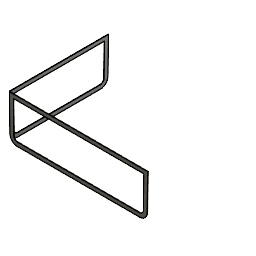
Hardcase_Gridfinity_Perimeter_Template (Autodesk Fusion 360 design; units mm, degrees)
part number: 2026-06-07-12-46-21-203
part number: 2026-06-07-12-46-21-213
Autodesk Fusion 360 part; units mm, degrees
sketch "FRONT" plane through (0, 0, 0) normal (0, 0, 1) x (1, 0, 0)
  line L0 (0, 0) -> (0, 110) construction
  line L1 (0, 110) -> (1.5933, 18.7175)
  line L2 (0, 110) -> (103.8151, 110) construction
  line L3 (20.6404, 0) -> (329.3596, 0)
  line L4 (350, 0) -> (350, 110) construction
  line L5 (350, 110) -> (348.4067, 18.7175)
  line L6 (350, 110) -> (486.4264, 110) construction
  line L7 (350, 110) -> (375.4, 110)
  line L8 (375.4, 110) -> (375.4, -25.4)
  line L9 (375.4, -25.4) -> (-25.4, -25.4)
  line L10 (-25.4, -25.4) -> (-25.4, 110)
  line L11 (-25.4, 110) -> (0, 110)
  arc A0 (1.5933, 18.7175) -> (20.6404, 0) centre (20.6404, 19.05) ccw
  arc A1 (329.3596, 0) -> (348.4067, 18.7175) centre (329.3596, 19.05) ccw
  line L12 (350, 110) -> (0, 110)
  line L13 (339.8239, 100) -> (10.1761, 100)
  line L14 (10.1761, 100) -> (11.5918, 18.8921)
  arc A2 (11.5918, 18.8921) -> (20.6404, 10) centre (20.6404, 19.05) ccw
  line L15 (20.6404, 10) -> (329.3596, 10)
  arc A3 (329.3596, 10) -> (338.4082, 18.8921) centre (329.3596, 19.05) ccw
  line L16 (339.8239, 100) -> (338.4082, 18.8921)
  dimension "d15" = 110
  dimension "d16" = 89
  dimension "d17" = 350
  dimension "d18" = 110
  dimension "d19" = 91
  dimension "d20" = 25.4
  dimension "d21" = 135.4
  dimension "d22" = 400.8
  dimension "d23" = 135.4
  dimension "d24" = 19.05
  constraint coincident L0.start origin
  constraint vertical L0
  constraint horizontal L2
  constraint perpendicular L0 L3
  constraint perpendicular L3 L4
  constraint horizontal L6
  constraint perpendicular L4 L7
  constraint perpendicular L6 L8
  constraint perpendicular L8 L9
  constraint perpendicular L9 L10
  constraint coincident L0.start L3
  constraint tangent L1 A0
  constraint tangent L3 A0
  constraint coincident L4.start L3
  constraint tangent L3 A1
  constraint tangent L5 A1
  constraint equal A0 A1
  measures "d15" distance of L0.start L0.end
  measures "d16" angle of L1 L2
  measures "d17" distance of L0.start L4.start
  measures "d18" distance of L4.start L4.end
  measures "d19" angle of L5 L6
  measures "d20" distance of L4.end L7.end
  measures "d21" distance of L7.end L8.end
  measures "d22" distance of L8.end L9.end
  measures "d23" distance of L9.end L10.end
  measures "d24" radius of A0
sketch "SIDE" plane through (0, 0, 0) normal (1, 0, 0) x (0, 0, -1)
  line L0 (0, 0) -> (0, 110) construction
  line L1 (20.6404, 0) -> (229.3596, 0)
  line L2 (250, 0) -> (250, 110) construction
  line L3 (250, 110) -> (248.4067, 18.7175)
  line L4 (250, 110) -> (374.6664, 110) construction
  line L5 (0, 110) -> (1.5933, 18.7175)
  line L6 (0, 110) -> (107.9664, 110) construction
  line L7 (0, 110) -> (-25.4, 110)
  line L8 (-25.4, 110) -> (-25.4, -25.4)
  line L9 (-25.4, -25.4) -> (275.4, -25.4)
  line L10 (275.4, -25.4) -> (275.4, 110)
  line L11 (275.4, 110) -> (250, 110)
  arc A0 (1.5933, 18.7175) -> (20.6404, 0) centre (20.6404, 19.05) ccw
  arc A1 (229.3596, 0) -> (248.4067, 18.7175) centre (229.3596, 19.05) ccw
  line L12 (250, 110) -> (0, 110)
  arc A2 (11.5918, 18.8921) -> (20.6404, 10) centre (20.6404, 19.05) ccw
  line L13 (20.6404, 10) -> (229.3596, 10)
  arc A3 (229.3596, 10) -> (238.4082, 18.8921) centre (229.3596, 19.05) ccw
  line L14 (239.8239, 100) -> (238.4082, 18.8921)
  line L15 (239.8239, 100) -> (10.1761, 100)
  line L16 (10.1761, 100) -> (11.5918, 18.8921)
  dimension "d151" = 110
  dimension "d152" = 250
  dimension "d153" = 110
  dimension "d154" = 91
  dimension "d155" = 89
  dimension "d156" = 25.4
  dimension "d157" = 135.4
  dimension "d158" = 300.8
  dimension "d159" = 135.4
  dimension "d160" = 25.4
  dimension "d161" = 19.05
  constraint coincident L0.start origin
  constraint vertical L0
  constraint perpendicular L0 L1
  constraint perpendicular L1 L2
  constraint horizontal L4
  constraint horizontal L6
  constraint perpendicular L0 L7
  constraint perpendicular L7 L8
  constraint perpendicular L8 L9
  constraint perpendicular L9 L10
  constraint perpendicular L10 L11
  constraint coincident L0.start L1
  constraint tangent L1 A0
  constraint tangent L5 A0
  constraint coincident L2.start L1
  constraint tangent L1 A1
  constraint tangent L3 A1
  constraint equal A0 A1
  measures "d151" distance of L0.start L0.end
  measures "d152" distance of L0.start L2.start
  measures "d153" distance of L2.start L2.end
  measures "d154" angle of L3 L4
  measures "d155" angle of L5 L6
  measures "d156" distance of L0.end L7.end
  measures "d157" distance of L7.end L8.end
  measures "d158" distance of L8.end L9.end
  measures "d159" distance of L9.end L10.end
  measures "d160" distance of L10.end L2.end
  measures "d161" radius of A0
extrude "Extrude36" add sketch "SIDE" against normal blind 1 contours L1 L3 L5 A0 A1 L12 makes body 1
extrude "Extrude37" add sketch "FRONT" along normal blind 1 separate body contours L1 L3 L5 A0 A1 L12 makes body 2
copy_body "Body->Comp8" bodies 1 removing the originals makes body 3 in component "Side Test"
copy_body "Body->Comp9" bodies 2 removing the originals makes body 4 in component "Front Test"
ref_plane "WorkPlane3" through (175, 0, 0) normal (1, 0, 0) x (0, 1, 0)
split "Split1" [suppressed] in component "Front Test"
component "Side Test" placed x (1, 0, 0) y (0, 1, 0) z (0, 0, 1) at (0, 0, 0)
component "Front Test" placed x (1, 0, 0) y (0, 1, 0) z (0, 0, 1) at (0, 0, 0)
equation "Overall_HT = 110 mm"
equation "OVERALL_LENGTH = 350 mm"
equation "OVERALL_WIDTH = 250 mm"
equation "BOTTOM_CORNER_RADIUS = 0.75 in"
equation "SIDE_WALL_TAPER = 1 deg"
equation "FRONT_WALL_TAPER = 1 deg"
equation "GRID_SPACING = 15 mm"
equation "d15 = Overall_HT"
equation "d16 = 90 deg - SIDE_WALL_TAPER"
equation "d17 = OVERALL_LENGTH"
equation "d18 = Overall_HT"
equation "d19 = 90 deg + SIDE_WALL_TAPER"
equation "d21 = Overall_HT + 1 in"
equation "d22 = OVERALL_LENGTH + 2 in"
equation "d23 = Overall_HT + 1 in"
equation "d24 = BOTTOM_CORNER_RADIUS"
equation "d151 = Overall_HT"
equation "d152 = OVERALL_WIDTH"
equation "d153 = Overall_HT"
equation "d154 = 90 deg + FRONT_WALL_TAPER"
equation "d155 = 90 deg - FRONT_WALL_TAPER"
equation "d156 = 1\""
equation "d157 = Overall_HT + 1\""
equation "d158 = OVERALL_WIDTH + 2\""
equation "d159 = Overall_HT + 1\""
equation "d160 = 1\""
equation "d161 = BOTTOM_CORNER_RADIUS"
equation "d571 = -TEST_OFFSET"
equation "d572 = -TEST_OFFSET"
equation "TEST_THICK = 1 mm"
equation "d574 = -TEST_THICK"
equation "d576 = TEST_THICK"
equation "TEST_OFFSET = 10 mm"
equation "d579 = OVERALL_LENGTH / 2"
named bodies: "Side Test", "Front Test", "Front Test (1)"
